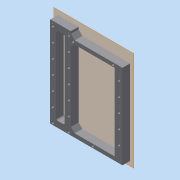
# Autodesk Inventor part: 09_Opentrons_Microscope_Baseplate
Saved by Autodesk Inventor 2019.4 (Build 234330000, 330)
## iProperties
Created: 2020-11-23
Part Number: 09_Opentrons_Microscope_Baseplate
Material: Generic
Document SubType Name: Modeling
Designer: diederichbenedict
Density: 1 g/cm^3
Appearance: Default
Author: diederichbenedict
Autodesk Inventor part; units mm, degrees
ref_plane "YZ Plane" through (0, 0, 0) normal (1, 0, 0) x (0, 1, 0)
ref_plane "XZ Plane" through (0, 0, 0) normal (0, 1, 0) x (-1, 0, 0)
ref_plane "XY Plane" through (0, 0, 0) normal (0, 0, 1) x (1, 0, 0)
ref_plane "Work Plane1" through (0, 0, 0) normal (0, 0, 1) x (1, 0, 0)
sketch "Sketch1" plane through (0, 0, 0) normal (0, 0, 1) x (1, 0, 0)
  circle A0 centre (152.1, -76.5) radius 1.45 projected
  circle A1 centre (152.1, 33) radius 1.45 projected
  circle A2 centre (152.1, 69.5) radius 1.45 projected
  circle A3 centre (152.1, -3.5) radius 1.45 projected
  circle A4 centre (152.1, -40) radius 1.45 projected
  line L0 (142.1, -108) -> (37.5, -108) projected
  line L1 (27.5, -98) -> (37.5, -108) projected
  line L2 (27.5, -98) -> (27.5, 82.5) projected
  line L3 (37.5, 92.5) -> (27.5, 82.5) projected
  line L4 (142.1, 92.5) -> (37.5, 92.5) projected
  line L5 (142.1, 92.5) -> (142.1, -108) projected
  circle A5 centre (136.5542, 97.5) radius 1.45 projected
  circle A6 centre (32.0458, 97.5) radius 1.45 projected
  circle A7 centre (83.8, -113) radius 1.45 projected
  line L6 (-25.5, -118) -> (162.1, -118) projected
  line L7 (162.1, -118) -> (162.1, 102.5) projected
  line L8 (37.5, 102.5) -> (162.1, 102.5) projected
  line L9 (27.5, 112.5) -> (37.5, 102.5) projected
  line L10 (27.5, 112.5) -> (27.5, 116) projected
  arc A8 (27.5, 116) -> (25.5, 118) centre (25.5, 116) ccw projected
  line L11 (25.5, 118) -> (-25.5, 118) projected
  arc A9 (-25.5, 118) -> (-27.5, 116) centre (-25.5, 116) ccw projected
  line L12 (-27.5, 116) -> (-27.5, -116) projected
  arc A10 (-27.5, -116) -> (-25.5, -118) centre (-25.5, -116) ccw projected
  circle A11 centre (-21, 106) radius 1.45 projected
  circle A12 centre (-21, 69.5) radius 1.45 projected
  circle A13 centre (-21, 33) radius 1.45 projected
  circle A14 centre (-21, -3.5) radius 1.45 projected
  circle A15 centre (-21, -40) radius 1.45 projected
  circle A16 centre (-21, -113) radius 1.45 projected
  circle A17 centre (21, -113) radius 1.45 projected
  circle A18 centre (21, -40) radius 1.45 projected
  circle A19 centre (21, -3.5) radius 1.45 projected
  circle A20 centre (21, 33) radius 1.45 projected
  circle A21 centre (21, 69.5) radius 1.45 projected
  circle A22 centre (21, 106) radius 1.45 projected
  arc A23 (-6.5, 102) -> (-11.5, 97) centre (-6.5, 97) ccw projected
  line L13 (-6.5, 102) -> (6.5, 102) projected
  arc A24 (11.5, 97) -> (6.5, 102) centre (6.5, 97) ccw projected
  line L14 (11.5, 97) -> (11.5, -97) projected
  arc A25 (6.5, -102) -> (11.5, -97) centre (6.5, -97) ccw projected
  line L15 (6.5, -102) -> (-6.5, -102) projected
  arc A26 (-11.5, -97) -> (-6.5, -102) centre (-6.5, -97) ccw projected
  line L16 (-11.5, -97) -> (-11.5, 97) projected
  circle A27 centre (21, -76.5) radius 1.45 projected
  circle A28 centre (-21, -76.5) radius 1.45 projected
  circle A29 centre (21, 111.5) radius 1.45 projected
  circle A30 centre (-21, 111.5) radius 1.45 projected
  point P0 (0, 0)
extrude "Extrusion1" add sketch "Sketch1" along normal blind 10
sketch "Sketch2" plane through (0, 0, 10) normal (0, 0, 1) x (1, 0, 0)
  line L0 (37.5, -108) -> (27.5, -98) projected
  line L1 (27.5, -98) -> (27.5, 82.5) projected
  line L2 (27.5, 82.5) -> (37.5, 92.5) projected
  line L3 (37.5, 92.5) -> (142.1, 92.5) projected
  line L4 (142.1, 92.5) -> (142.1, -108) projected
  line L5 (142.1, -108) -> (37.5, -108) projected
  line L6 (-6.5, 102) -> (6.5, 102) projected
  arc A0 (11.5, 97) -> (6.5, 102) centre (6.5, 97) ccw projected
  line L7 (11.5, 97) -> (11.5, -97) projected
  arc A1 (6.5, -102) -> (11.5, -97) centre (6.5, -97) ccw projected
  line L8 (6.5, -102) -> (-6.5, -102) projected
  arc A2 (-11.5, -97) -> (-6.5, -102) centre (-6.5, -97) ccw projected
  line L9 (-11.5, -97) -> (-11.5, 97) projected
  arc A3 (-6.5, 102) -> (-11.5, 97) centre (-6.5, 97) ccw projected
  circle A4 centre (-21, 111.5) radius 1.45 projected
  circle A5 centre (21, 111.5) radius 1.45 projected
  circle A6 centre (-21, -76.5) radius 1.45 projected
  circle A7 centre (21, -76.5) radius 1.45 projected
  circle A8 centre (21, 106) radius 1.45 projected
  circle A9 centre (21, 69.5) radius 1.45 projected
  circle A10 centre (21, 33) radius 1.45 projected
  circle A11 centre (21, -3.5) radius 1.45 projected
  circle A12 centre (21, -40) radius 1.45 projected
  circle A13 centre (21, -113) radius 1.45 projected
  circle A14 centre (-21, -113) radius 1.45 projected
  circle A15 centre (-21, -40) radius 1.45 projected
  circle A16 centre (-21, -3.5) radius 1.45 projected
  circle A17 centre (-21, 33) radius 1.45 projected
  circle A18 centre (-21, 69.5) radius 1.45 projected
  circle A19 centre (-21, 106) radius 1.45 projected
  circle A20 centre (83.8, -113) radius 1.45 projected
  circle A21 centre (32.0458, 97.5) radius 1.45 projected
  circle A22 centre (136.5542, 97.5) radius 1.45 projected
  circle A23 centre (152.1, -40) radius 1.45 projected
  circle A24 centre (152.1, -3.5) radius 1.45 projected
  circle A25 centre (152.1, 69.5) radius 1.45 projected
  circle A26 centre (152.1, 33) radius 1.45 projected
  circle A27 centre (152.1, -76.5) radius 1.45 projected
  line L10 (-25.5, -118) -> (162.1, -118) projected
  line L11 (162.1, -118) -> (162.1, 102.5) projected
  line L12 (162.1, 102.5) -> (37.5, 102.5) projected
  line L13 (37.5, 102.5) -> (27.5, 112.5) projected
  line L14 (27.5, 112.5) -> (27.5, 116) projected
  arc A28 (27.5, 116) -> (25.5, 118) centre (25.5, 116) ccw projected
  line L15 (25.5, 118) -> (-25.5, 118) projected
  arc A29 (-25.5, 118) -> (-27.5, 116) centre (-25.5, 116) ccw projected
  line L16 (-27.5, 116) -> (-27.5, -116) projected
  arc A30 (-27.5, -116) -> (-25.5, -118) centre (-25.5, -116) ccw projected
  point P0 (0, 0)
  point P1 (30.8984, 98.3623)
  point P2 (153.55, -76.5)
hole "Hole1" at (83.8, -113, 10) at (21, -113, 10) at (-21, -113, 10) at (-21, -76.5, 10) at (-21, -40, 10) at (-21, -3.5, 10) at (-21, 33, 10) at (-21, 69.5, 10) at (-21, 106, 10) at (21, 106, 10) at (32.0458, 97.5, 10) at (21, 69.5, 10) at (21, 33, 10) at (21, -3.5, 10) at (21, -40, 10) at (21, -76.5, 10) at (152.1, -76.5, 10) at (152.1, -40, 10) at (152.1, -3.5, 10) at (152.1, 33, 10) at (152.1, 69.5, 10) at (136.5542, 97.5, 10) direction (0, 0, -1) diameter 2.9 end through all counterbore diameter 7 counterbore depth 7
body "Solid1"
